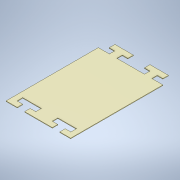
# Autodesk Inventor part: TopCoverLayer
Saved by Autodesk Inventor 2020 (Build 240168000, 168)
## iProperties
Created: 2021-01-27
Part Number: TopCoverLayer
Material: Acrylic
Document SubType Name: Modeling
Designer: abij996
Density: 1.188 g/cm^3
Appearance: Smooth - Ash
Author: abij996
Autodesk Inventor part; units mm, degrees
ref_plane "YZ Plane" through (0, 0, 0) normal (1, 0, 0) x (0, 1, 0)
ref_plane "XZ Plane" through (0, 0, 0) normal (0, 1, 0) x (-1, 0, 0)
ref_plane "XY Plane" through (0, 0, 0) normal (0, 0, 1) x (1, 0, 0)
sketch "Sketch1" plane through (0, 0, 0) normal (0, 1, 0) x (-1, 0, 0)
  line L0 (-348.8673, 325.8519) -> (-348.8673, -174.1481)
  line L1 (1.1327, -174.1481) -> (1.1327, 325.8519)
  line L2 (-98.8673, -174.1481) -> (-98.8673, -204.1481)
  line L3 (-58.8673, -203.2202) -> (-58.8673, -174.1481)
  line L4 (-128.8673, -204.1481) -> (-128.8673, -234.1481)
  line L5 (-128.8673, -234.1481) -> (-28.8673, -234.1481)
  line L6 (-28.8673, -234.1481) -> (-28.8673, -203.2202)
  line L7 (-58.8673, -174.1481) -> (1.1327, -174.1481)
  line L8 (-28.8673, -203.2202) -> (-58.8673, -203.2202)
  line L9 (-98.8673, -204.1481) -> (-128.8673, -204.1481)
  line L10 (-99.6673, 325.8519) -> (-99.6673, 296.2519)
  line L11 (-59.2673, 296.2519) -> (-59.2673, 325.8519)
  line L12 (-130.0673, 296.2519) -> (-130.0673, 265.4519)
  line L13 (-130.0673, 265.4519) -> (-28.8673, 265.4519)
  line L14 (-28.8673, 265.4519) -> (-28.8673, 296.2519)
  line L15 (-28.8673, 296.2519) -> (-59.2673, 296.2519)
  line L16 (-99.6673, 296.2519) -> (-130.0673, 296.2519)
  line L17 (1.1327, 325.8519) -> (-59.2673, 325.8519)
  line L18 (-320.4673, 296.2519) -> (-320.4673, 265.4519)
  line L19 (-320.4673, 265.4519) -> (-219.2673, 265.4519)
  line L20 (-219.2673, 265.4519) -> (-219.2673, 296.2519)
  line L21 (-290.0673, 325.8519) -> (-290.0673, 296.2519)
  line L22 (-249.6673, 296.2519) -> (-249.6673, 325.8519)
  line L23 (-318.8673, -204.1481) -> (-318.8673, -234.1481)
  line L24 (-318.8673, -234.1481) -> (-218.8673, -234.1481)
  line L25 (-218.8673, -234.1481) -> (-218.8673, -204.1481)
  line L26 (-288.8673, -174.1481) -> (-288.8673, -204.1481)
  line L27 (-248.8673, -204.1481) -> (-248.8673, -174.1481)
  line L28 (-99.6673, 325.8519) -> (-249.6673, 325.8519)
  line L29 (-290.0673, 325.8519) -> (-348.8673, 325.8519)
  line L30 (-219.2673, 296.2519) -> (-249.6673, 296.2519)
  line L31 (-290.0673, 296.2519) -> (-320.4673, 296.2519)
  line L32 (-348.8673, -174.1481) -> (-288.8673, -174.1481)
  line L33 (-248.8673, -174.1481) -> (-98.8673, -174.1481)
  line L34 (-218.8673, -204.1481) -> (-248.8673, -204.1481)
  line L35 (-288.8673, -204.1481) -> (-318.8673, -204.1481)
  point P0 (0, 0)
  dimension "d0" = 500
  dimension "d1" = 350
  dimension "d5" = 100
  dimension "d6" = 40.4
  dimension "d7" = 40
  dimension "d8" = 30
  dimension "d9" = 30.4
  dimension "d11" = 30
  dimension "d15" = 30
  dimension "d20" = 30
  dimension "d30" = 500
  dimension "d33" = 40.4
  dimension "d35" = 30.4
  dimension "d36" = 29.6
  dimension "d37" = 29.6
  dimension "d38" = 30.8
  dimension "d39" = 30.4
  dimension "d40" = 30.4
  dimension "d41" = 30.8
  dimension "d42" = 30.8
  dimension "d43" = 29.6
  constraints: 72 end point, 26 parallel, 11 horizontal, 11 perpendicular, 3 collinear
  measures "d0" distance of L1.start L1.end
  measures "d1" distance of L0.end L1.start
  measures "d5" distance of L4.end L5.end
  measures "d6" distance between parallel lines of L10 L11
  measures "d7" distance between parallel lines of L2 L3
  measures "d8" distance of L6.end L3.start
  measures "d9" distance between parallel lines of L11 L14
  measures "d11" distance of L2.start L2.end
  measures "d15" distance between parallel lines of L1 L6
  measures "d20" distance of L4.start L4.end
  measures "d30" distance of L0.start L0.end
  measures "d33" distance between parallel lines of L21 L22
  measures "d35" distance between parallel lines of L12 L10
  measures "d36" distance between parallel lines of L28 L16
  measures "d37" distance between parallel lines of L15 L17
  measures "d38" distance of L13.end L14.end
  measures "d39" distance between parallel lines of L22 L20
  measures "d40" distance between parallel lines of L21 L18
  measures "d41" distance of L19.end L20.end
  measures "d42" distance of L18.start L18.end
  measures "d43" distance between parallel lines of L29 L31
extrude "Extrusion2" add sketch "Sketch1" against normal blind 3
body "Solid2"
